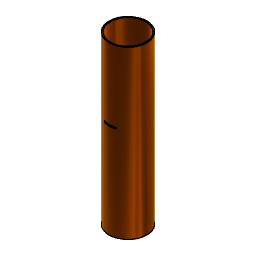
Motor mount tube v8 (Autodesk Fusion 360 design; units mm, degrees)
Autodesk Fusion 360 part; units mm, degrees
note: some values were not read from the file. Set by a fixed rule: which sketch regions a step uses.
sketch "Sketch1" plane through (0, 0, 0) normal (0, 0, 1) x (1, 0, 0)
  circle A0 centre (0, 0) radius 15
  circle A1 centre (0, 0) radius 16
  dimension "d1" = 30
  dimension "d2" = 32
  constraint coincident A0.centre A1.centre
  measures "d1" diameter of A0
  measures "d2" diameter of A1
extrude "Extrude1" add sketch "Sketch1" along normal blind 140
sketch "Sketch2" plane through (0, 0, 0) normal (0, 1, 0) x (1, 0, 0)
  line L0 (0, 0) -> (0, -78.88) construction
  line L1 (5, -79.88) -> (-5, -79.88)
  line L2 (-5, -79.88) -> (-5, -78.88)
  line L3 (5, -78.88) -> (5, -79.88)
  line L4 (5, -79.88) -> (0, -78.88) construction
  line L5 (-5, -79.88) -> (0, -78.88) construction
  line L6 (-5, -79.88) -> (5, -79.88)
  line L7 (5, -79.88) -> (5, -78.88)
  line L8 (5, -78.88) -> (-5, -78.88)
  line L9 (-5, -78.88) -> (-5, -79.88)
  point P0 (0, -78.88)
  dimension "d5" = 78.88
  constraint coincident L0.start origin
  constraint vertical L0
  constraint horizontal L1
  constraint perpendicular L1 L2
  constraint parallel L2 L3
  constraint coincident L4 P0
  constraint coincident L5 P0
  constraint coincident P0 L0.end
  constraint horizontal L6
  constraint vertical L7
  constraint horizontal L8
  constraint vertical L9
  measures "d5" distance of L0.start P0
extrude "Extrude2" cut sketch "Sketch2" along normal through all and the other way through all
sketch "Sketch3" plane through (0, 0, 0) normal (0, 0, -1) x (1, 0, 0)
  circle A0 centre (0, 0) radius 15
  circle A1 centre (0, 0) radius 16
  circle A2 centre (0, 0) radius 16
  circle A3 centre (0, 0) radius 15
  constraint coincident A0.centre A1.centre
extrude "Extrude3" add sketch "Sketch3" along normal blind 1.25
equation "d5 = 80 mm - 1.12 mm"
